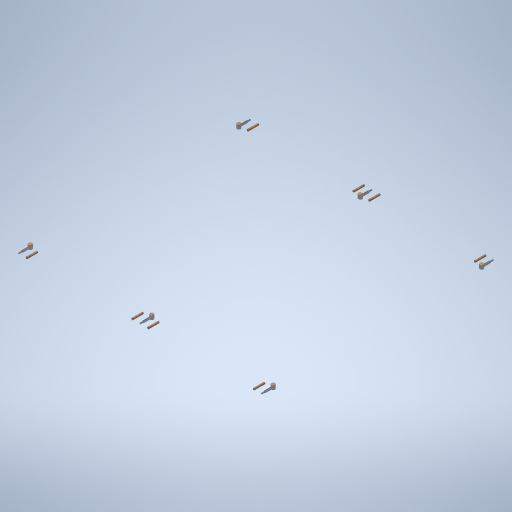
# Autodesk Inventor part: REC_04
Saved by Autodesk Inventor 2024.3 (Build 283343000, 343)
## iProperties
RuleStatus: InUse
Created: 2014-05-08
Part Number: REC_04
Material: Generic
Document SubType Name: Modeling
Designer: SauliusD
Density: 1 g/cm^3
Appearance: Default
Description: Pillar Board & 2 Nestled Boards from Sides Minifixes-04
AfterDocNew0: Fire Form
Author: SauliusD
Autodesk Inventor part; units mm, degrees
sketch "Sketch2" plane through (0, 0, 0) normal (0, 0, 1) x (1, 0, 0)
  line L0 (-178.2411, -758.1253) -> (817.7589, -758.1253)
  line L1 (817.7589, -758.1253) -> (817.7589, 161.8747)
  line L2 (817.7589, 161.8747) -> (-178.2411, 161.8747)
  line L3 (-178.2411, 161.8747) -> (-178.2411, -758.1253)
  point P0 (319.7589, 161.8747)
  point P1 (817.7589, -298.1253)
  constraints: 8 end point, 2 midpoint, 2 parallel, 1 horizontal, 1 perpendicular
ref_plane "Work Plane1" through (0, 0, -9) normal (0, 0, 1) x (1, 0, 0)
sketch "Sketch3" plane through (0, 0, -9) normal (0, 0, 1) x (1, 0, 0)
  line L0 (-178.2411, 161.8747) -> (-178.2411, -758.1253) construction
  line L1 (817.7589, 161.8747) -> (-178.2411, 161.8747) construction
  line L2 (817.7589, -758.1253) -> (817.7589, 161.8747) construction
  line L3 (-176.2411, 161.8747) -> (-172.2411, 161.8747)
  line L4 (-172.2411, 161.8747) -> (-172.2411, 127.8747)
  line L5 (-172.2411, 127.8747) -> (-176.2411, 127.8747)
  line L6 (-176.2411, 127.8747) -> (-176.2411, 161.8747)
  line L7 (-176.2411, 161.8747) -> (-173.7411, 161.8747)
  line L8 (-173.7411, 161.8747) -> (-173.7411, 174.8747)
  line L9 (-173.7411, 174.8747) -> (-176.2411, 174.8747)
  line L10 (-176.2411, 174.8747) -> (-176.2411, 161.8747)
  line L11 (319.7589, 161.8747) -> (319.7589, 132.7708) construction
  line L12 (815.7589, 127.8747) -> (815.7589, 161.8747)
  point P0 (0, 0)
  dimension "d5" = 8
  dimension "d7" = 5
  dimension "d8" = 13
  dimension "Dist_Between_Planes" = 996
  dimension "Distance_between_Axis" = 992
  constraints: 20 end point, 5 parallel, 2 horizontal, 2 perpendicular, 2 symmetric about line, 1 collinear, 1 midpoint, 1 vertical alignment
  measures "d5" diameter of L4 L6
  measures "d7" diameter of L8 L10
  measures "d8" distance of L7.end L8.end
  measures "Dist_Between_Planes" distance of L1.start L0.start
  measures "Distance_between_Axis" distance between parallel lines of L6 L12
revolve "Minifix Revolve" add sketch "Sketch3" angle 360 about axis through (-176.2411, 174.8747, -9) along (0, -1, 0)
sketch "Sketch4" plane through (0, 0, -9) normal (0, 0, 1) x (1, 0, 0)
  line L0 (-180.2411, 127.8747) -> (-172.2411, 127.8747) construction
  circle A0 centre (-176.2411, 127.8747) radius 7.5
  point P0 (0, 0)
  dimension "d10" = 15
  constraints: 1 centre point, 1 midpoint
  measures "d10" diameter of A0
extrude "Minifix Extrude" add sketch "Sketch4" along normal up to surface (9 mm away)
extrude "Minifix extrude 2" add sketch "Sketch4" against normal blind 6
ref_plane "Work Plane2" through (319.7589, 161.8747, 0) normal (1, 0, 0) x (0, 1, 0)
ref_plane "Work Plane3" through (817.7589, -298.1253, 0) normal (0, 1, 0) x (-1, 0, 0)
sketch "Sketch5" plane through (0, 0, -9) normal (0, 0, 1) x (1, 0, 0)
  line L0 (-176.2411, 361.4747) -> (-176.2411, -944.7253) construction
  line L1 (-144.2411, 174.8747) -> (-144.2411, 131.8747)
  line L2 (-144.2411, 174.8747) -> (-140.2411, 174.8747)
  line L3 (-140.2411, 174.8747) -> (-140.2411, 131.8747)
  line L4 (-140.2411, 131.8747) -> (-144.2411, 131.8747)
  line L5 (-178.7411, 174.8747) -> (-173.7411, 174.8747) construction
  line L6 (-180.2411, 161.8747) -> (-172.2411, 161.8747) construction
  point P0 (0, 0)
  dimension "Dowel_D" = 8
  dimension "Dowel_Drill_Depth" = 30
  dimension "d17" = 32
  constraints: 8 end point, 2 parallel, 2 perpendicular, 1 collinear
  measures "Dowel_D" diameter of L3 L1
  measures "Dowel_Drill_Depth" distance between parallel lines of L4 L6
  measures "d17" distance from line of L1.start L0
revolve "Dowel Revolve" add sketch "Sketch5" angle 360 about axis through (-144.2411, 174.8747, -9) along (0, -1, 0) separate body
mirror "Mirror1" about plane through (319.7589, 161.8747, 0) normal (1, 0, 0) of "Minifix Extrude", "Minifix Revolve", "Dowel Revolve", "Minifix extrude 2" bodies 1
sketch "Sketch6" plane through (0, 0, -9) normal (0, 0, 1) x (1, 0, 0)
  point P0 (0, 0)
sketch "Sketch7" plane through (0, 0, -9) normal (0, 0, 1) x (1, 0, 0)
  line L0 (319.7589, 361.4747) -> (319.7589, -944.7253) construction
  line L1 (322.2589, 161.8747) -> (319.7589, 161.8747)
  line L2 (319.7589, 161.8747) -> (319.7589, 174.8747)
  line L3 (319.7589, 174.8747) -> (322.2589, 174.8747)
  line L4 (322.2589, 174.8747) -> (322.2589, 161.8747)
  line L5 (319.7589, 161.8747) -> (323.7589, 161.8747)
  line L6 (323.7589, 161.8747) -> (323.7589, 127.8747)
  line L7 (323.7589, 127.8747) -> (319.7589, 127.8747)
  line L8 (319.7589, 127.8747) -> (319.7589, 161.8747)
  line L9 (-178.7411, 174.8747) -> (-173.7411, 174.8747) construction
  line L10 (-180.2411, 161.8747) -> (-172.2411, 161.8747) construction
  point P0 (0, 0)
  point P1 (319.7589, -944.7253)
  dimension "d19" = 34
  dimension "d20" = 5
  dimension "d21" = 8
  constraints: 16 end point, 4 parallel, 2 collinear, 2 horizontal, 2 perpendicular, 1 vertical, 1 other
  measures "d19" distance of L5.end L6.end
  measures "d20" diameter of L4 L2
  measures "d21" diameter of L6 L2
revolve "Center minixix Revolution" add sketch "Sketch7" angle 360 about axis through (319.7589, 161.8747, -9) along (0, 1, 0) separate body
sketch "Sketch8" plane through (0, 0, -9) normal (0, 0, 1) x (1, 0, 0)
  circle A0 centre (319.7589, 127.8747) radius 7.5
  line L0 (323.7589, 127.8747) -> (319.7589, 127.8747) construction
  point P0 (0, 0)
  dimension "d23" = 15
  constraints: 1 centre point, 1 coincident
  measures "d23" diameter of A0
extrude "Center minixix Extrusion 1" add sketch "Sketch8" along normal up to surface (9 mm away) bodies 3
extrude "Center minixix Extrusion 2" add sketch "Sketch8" against normal up to surface (6 mm away) bodies 3
ref_plane "Work Plane4" through (-178.2411, 161.8747, 0) normal (0, 1, 0) x (-1, 0, 0)
mirror "Mirror2" about plane through (817.7589, -298.1253, 0) normal (0, 1, 0) of "Minifix Extrude", "Minifix Revolve", "Dowel Revolve", "Minifix extrude 2", "Mirror1" bodies 1
mirror "Mirror Center" about plane through (817.7589, -298.1253, 0) normal (0, 1, 0) of "Center minixix Revolution", "Center minixix Extrusion 1", "Center minixix Extrusion 2" bodies 3
sketch "Sketch9" plane through (-176.2411, 127.8747, 0) normal (0, 0, 1) x (1, 0, 0)
  circle A0 centre (0, 0) radius 7.5 projected
  point P0 (176.2411, -127.8747)
extrude "Side Cover Cap Extrusion" add sketch "Sketch9" along normal blind 2 separate body
fillet "Side Cover Cap Fillet" radius 1.6 1 edges at (-183.7411, 127.8747, 2)
mirror "Mirror3" about plane through (319.7589, 161.8747, 0) normal (1, 0, 0) of "Side Cover Cap Extrusion", "Side Cover Cap Fillet" bodies 4
mirror "Mirror4" about plane through (817.7589, -298.1253, 0) normal (0, 1, 0) of "Side Cover Cap Extrusion", "Side Cover Cap Fillet", "Mirror3" bodies 4
sketch "Sketch10" plane through (0, 0, 0) normal (0, 0, 1) x (1, 0, 0)
  circle A0 centre (319.7589, 127.8747) radius 7.5
  line L0 (817.7589, 161.8747) -> (-178.2411, 161.8747) projected
  point P0 (18.2411, -127.8747)
  point P1 (319.7589, 161.8747)
  dimension "d42" = 34
  constraints: 1 centre point, 1 midpoint, 1 vertical alignment
  measures "d42" distance from line of L0 A0.centre
extrude "Center Cover Cap Extrusion" add sketch "Sketch10" along normal blind 2 separate body
fillet "Center Cover Cap Fillet" radius 1.6 1 edges at (312.2589, 127.8747, 2)
mirror "Mirror5" about plane through (817.7589, -298.1253, 0) normal (0, 1, 0) of "Center Cover Cap Extrusion", "Center Cover Cap Fillet" bodies 5
sketch "Sketch11" plane through (0, 0, -9) normal (0, 0, 1) x (1, 0, 0)
  line L0 (319.7589, 348.4747) -> (319.7589, -957.7253) construction
  line L1 (283.7589, -771.1253) -> (287.7589, -771.1253)
  line L2 (287.7589, -771.1253) -> (287.7589, -728.1253)
  line L3 (287.7589, -728.1253) -> (283.7589, -728.1253)
  line L4 (283.7589, -728.1253) -> (283.7589, -771.1253)
  line L5 (787.7589, -771.1253) -> (779.7589, -771.1253) construction
  line L6 (787.7589, -728.1253) -> (779.7589, -728.1253) construction
  point P0 (0, 0)
  dimension "d43" = 8
  dimension "d44" = 32
  constraints: 8 end point, 2 collinear, 2 parallel, 1 horizontal, 1 perpendicular
  measures "d43" diameter of L4 L2
  measures "d44" distance from line of L1.end L0
revolve "Center Dowel Revolve" add sketch "Sketch11" angle 360 about axis through (287.7589, -771.1253, -9) along (0, 1, 0) bodies 1
mirror "Mirror7" about plane through (319.7589, 161.8747, 0) normal (1, 0, 0) of "Center Dowel Revolve" bodies 1
mirror "Mirror8" about plane through (817.7589, -298.1253, 0) normal (0, 1, 0) of "Center Dowel Revolve", "Mirror7" bodies 1
equation "\"d23\" = d10"
equation "\"d38\" = d35"
equation "\"d20\" = d7"
equation "\"d21\" = d5"
equation "\"d43\" = Dowel_D"
equation "\"d44\" = Step"
equation "\"Step\" = 32"
equation "\"d35\" = 1.6"
